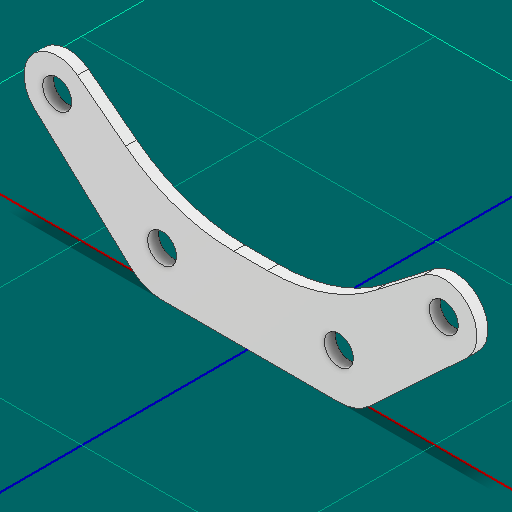
# Autodesk Inventor part: Hook Gusset Brace
Saved by Autodesk Inventor 2025 (Build 290162000, 162)
## iProperties
Created: 2024-10-13
Part Number: Hook Gusset Brace
Material: Acetal Resin, White
Document SubType Name: Modeling
Designer: Averey Ku
Density: 1.425 g/cm^3
Appearance: Smooth - White
Author: Averey Ku
Autodesk Inventor part; units mm, degrees
ref_plane "YZ Plane" through (0, 0, 0) normal (1, 0, 0) x (0, 1, 0)
ref_plane "XZ Plane" through (0, 0, 0) normal (0, 1, 0) x (-1, 0, 0)
ref_plane "XY Plane" through (0, 0, 0) normal (0, 0, 1) x (1, 0, 0)
sketch "Sketch1" plane through (0, 0, 0) normal (0, 0, 1) x (1, 0, 0)
  circle A0 centre (13.2036, 20.3187) radius 2.0955
  circle A1 centre (-12.1964, 20.3187) radius 2.0955
  line L0 (2.9057, 25.0812) -> (-1.8984, 25.0812)
  circle A2 centre (-27.2689, 31.9687) radius 2.0955
  arc A3 (-24.3564, 35.7368) -> (-30.5078, 28.4771) centre (-27.2689, 31.9687) ccw
  arc A4 (31.515, 28.4771) -> (25.3636, 35.7368) centre (28.2761, 31.9687) ccw
  circle A5 centre (28.2761, 31.9687) radius 2.0955
  line L1 (-24.3564, 35.7368) -> (-17.4317, 30.3845)
  line L2 (25.3636, 35.7368) -> (18.439, 30.3845)
  arc A6 (-17.4317, 30.3845) -> (-1.8984, 25.0812) centre (-1.8984, 50.4812) ccw
  arc A7 (2.9057, 25.0812) -> (18.439, 30.3845) centre (2.9057, 50.4812) ccw
  arc A8 (-16.5979, 15.5738) -> (-12.1964, 13.8467) centre (-12.1964, 20.3187) ccw
  arc A9 (13.2036, 13.8467) -> (17.6051, 15.5738) centre (13.2036, 20.3187) ccw
  line L3 (-12.1964, 13.8467) -> (13.2036, 13.8467)
  line L4 (-30.5078, 28.4771) -> (-16.5979, 15.5738)
  line L5 (17.6051, 15.5738) -> (31.515, 28.4771)
  point P0 (0, 0)
  point P1 (-12.1964, 25.0812)
  point P2 (17.4758, 18.214)
  point P3 (-16.4686, 18.214)
  dimension "d8" = 4.191
  dimension "d9" = 4.191
  dimension "d13" = 4.191
  dimension "d14" = 9.525
  dimension "d15" = 9.525
  dimension "d16" = 4.191
  dimension "d17" = 25.4
  constraints: 13 tangent, 12 end point, 12 point on circle, 10 centre point, 4 coincident, 1 equal radius, 1 horizontal, 2 other
  measures "d8" diameter of A1
  measures "d9" diameter of A0
  measures "d13" diameter of A2
  measures "d14" diameter of A3
  measures "d15" diameter of A4
  measures "d16" diameter of A5
  measures "d17" radius of A6
extrude "Extrusion1" add sketch "Sketch1" along normal blind 1.5875
body "Solid1"
